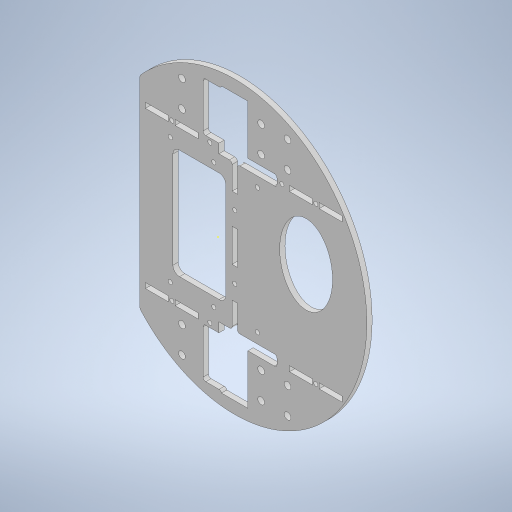
# Autodesk Inventor part: нижний эллипс тела
Saved by Autodesk Inventor 2023.1 (Build 271208000, 208)
## iProperties
Created: 2024-11-21
Part Number: нижний эллипс тела
Material: Типовые
Document SubType Name: Modeling
Designer: DELL
Density: 1 g/cm^3
Appearance: По умолчанию
Mass: 110.584 g
Surface Area: 588.358 cm^2
Volume: 110.584 cm^3
Author: DELL
Autodesk Inventor part; units mm, degrees
ref_plane "YZ Plane" through (0, 0, 0) normal (1, 0, 0) x (0, 1, 0)
ref_plane "XZ Plane" through (0, 0, 0) normal (0, 1, 0) x (-1, 0, 0)
ref_plane "XY Plane" through (0, 0, 0) normal (0, 0, 1) x (1, 0, 0)
sketch "Эскиз1" plane through (0, 0, 0) normal (0, 0, 1) x (1, 0, 0)
  ellipse E0 centre (12.6725, 0) end of major axis (12.6725, -110) minor radius 100
  dimension "d54" = 110
  dimension "d55" = 100
  constraints: 2 other
extrude "Выдавливание1" add sketch "Эскиз1" against normal blind 4
sketch "Эскиз5" plane through (0, 0, 0) normal (0, 0, 1) x (1, 0, 0)
  line L0 (10.6728, -60.9593) -> (10.6728, 60.5004) construction
  line L1 (14.6722, 60.5004) -> (14.6722, -60.9593) construction
  line L2 (14.6722, 60.5004) -> (10.6728, 60.5004)
  line L3 (14.6722, -60.9593) -> (10.6728, -60.9593)
  line L4 (10.6728, -35.9593) -> (14.6722, -35.9593)
  line L5 (10.6728, -12.5) -> (14.6722, -12.5)
  line L6 (10.6728, 12.5) -> (14.6722, 12.5)
  line L7 (10.6728, 35.5004) -> (14.6722, 35.5004)
  line L8 (10.6728, -12.5) -> (10.6728, 12.5)
  line L9 (14.6722, 12.5) -> (14.6722, -12.5)
  line L10 (14.6722, -12.5) -> (10.6728, 12.5) construction
  line L11 (10.6728, -60.9593) -> (10.6728, -35.9593)
  line L12 (14.6722, -35.9593) -> (14.6722, -60.9593)
  line L13 (14.6722, 35.5004) -> (14.6722, 60.5004)
  line L14 (10.6728, 35.5004) -> (10.6728, 60.5004)
  line L15 (14.6722, -35.9593) -> (10.6728, -12.5) construction
  circle A0 centre (12.6725, -24.2296) radius 1.575
  line L16 (14.6722, 12.5) -> (10.6728, 35.5004) construction
  circle A1 centre (12.6725, 24.0002) radius 1.575
  point P0 (0, 0)
  point P1 (12.6725, 0)
  point P2 (12.6725, 60.5004)
  point P3 (12.6725, 12.5)
  point P4 (12.6725, -12.5)
  point P5 (12.6725, 0)
  dimension "d35" = 25
  dimension "d36" = 25
  dimension "d37" = 25
  dimension "d38" = 3.15
  dimension "d39" = 3.15
  constraints: 34 end point, 8 point on line, 6 midpoint, 4 collinear, 4 perpendicular, 2 centre point, 2 parallel, 1 coincident
  measures "d35" distance from line of L1.end L4
  measures "d36" vertical distance of point (12.673, 60.5) L7.end
  measures "d37" distance of point (12.673, 12.5) point (12.673, -12.5)
  measures "d38" diameter of A0
  measures "d39" diameter of A1
extrude "Выдавливание3" cut sketch "Эскиз5" against normal blind 4
sketch "Эскиз7" plane through (0, 0, 0) normal (0, 0, 1) x (1, 0, 0)
  line L0 (4.1681, 100.5004) -> (8.7181, 100.5004) projected
  line L1 (2.6681, 94.4504) -> (2.6681, 99.0004) projected
  line L2 (2.6681, -99.4593) -> (2.6681, -94.9093) projected
  line L3 (8.7181, -100.9593) -> (4.1681, -100.9593) projected
  line L4 (2.6681, 100.5004) -> (22.6681, 100.5004)
  line L5 (22.6681, 100.5004) -> (22.6681, 60.5004)
  line L6 (22.6681, 60.5004) -> (2.6681, 60.5004)
  line L7 (2.6681, 60.5004) -> (2.6681, 100.5004)
  line L8 (2.6681, -100.9593) -> (22.6681, -100.9593)
  line L9 (22.6681, -100.9593) -> (22.6681, -60.9593)
  line L10 (22.6681, -60.9593) -> (2.6681, -60.9593)
  line L11 (2.6681, -60.9593) -> (2.6681, -100.9593)
  circle A0 centre (-7.3319, 80.5004) radius 5
  circle A1 centre (-7.3319, -80.9593) radius 5
  point P0 (0, 0)
  point P1 (2.6681, 80.5004)
  point P2 (2.6681, -80.9593)
  dimension "d44" = 20
  dimension "d45" = 40
  dimension "d46" = 20
  dimension "d47" = 40
  dimension "d48" = 10
  dimension "d49" = 10
  dimension "d50" = 10
  dimension "d51" = 10
  constraints: 16 end point, 4 parallel, 2 centre point, 2 horizontal, 2 midpoint, 2 perpendicular, 1 point on line
  measures "d44" distance of L5.end L6.end
  measures "d45" distance of L4.end L5.end
  measures "d46" distance of L10.end L9.end
  measures "d47" distance of L9.end L8.end
  measures "d48" diameter of A0
  measures "d49" diameter of A1
  measures "d50" distance of point (2.668, 80.5) A0.centre
  measures "d51" distance of point (2.668, -80.959) A1.centre
extrude "Выдавливание4" cut sketch "Эскиз7" against normal blind 4 contours L0 L4 L5 L6 L7 L1 | L2 L11 L10 L9 L8 L3
sketch "Эскиз8" plane through (0, 0, 0) normal (0, 0, 1) x (1, 0, 0)
  line L0 (-1.3319, 62.0004) -> (-1.3319, 99.0004) construction
  line L1 (-1.3319, 99.0004) -> (-9.3319, 99.0004) projected
  arc A0 (-9.3319, 99.0004) -> (-11.3319, 97.0004) centre (-9.3319, 97.0004) ccw projected
  line L2 (-11.3319, 97.0004) -> (-11.3319, 64.0004) projected
  line L3 (-9.3319, 62.0004) -> (-1.3319, 62.0004) projected
  arc A1 (-11.3319, 64.0004) -> (-9.3319, 62.0004) centre (-9.3319, 64.0004) ccw projected
  line L4 (-1.3319, -62.4593) -> (-9.3319, -62.4593) projected
  line L5 (-1.3319, -99.4593) -> (-1.3319, -62.4593) construction
  arc A2 (-9.3319, -62.4593) -> (-11.3319, -64.4593) centre (-9.3319, -64.4593) ccw projected
  line L6 (-11.3319, -64.4593) -> (-11.3319, -97.4593) projected
  line L7 (-9.3319, -99.4593) -> (-1.3319, -99.4593) projected
  arc A3 (-11.3319, -97.4593) -> (-9.3319, -99.4593) centre (-9.3319, -97.4593) ccw projected
  line L8 (-1.3319, -62.4593) -> (2.6681, -62.4593)
  line L9 (2.6681, -100.9593) -> (2.6681, -60.9593) construction
  line L10 (-1.3319, -99.4593) -> (2.6681, -99.4593)
  line L11 (2.6681, -60.9593) -> (2.6681, -100.9593) construction
  line L12 (2.6681, 60.5004) -> (2.6681, 100.5004) construction
  line L13 (-1.3319, 99.0004) -> (2.6681, 99.0004)
  line L14 (2.6681, 61.8452) -> (2.6681, 99.0004)
  line L15 (2.6681, -99.4593) -> (2.6681, -62.4593)
  line L16 (-1.3319, 62.0004) -> (2.6681, 62.0004)
  constraints: 12 end point, 4 point on line, 2 collinear, 2 horizontal, 1 parallel, 1 perpendicular
extrude "Выдавливание5" cut sketch "Эскиз8" against normal blind 10
fillet "Сопряжение1" radius 2 4 edges at (2.6681, -99.4593, -2) (2.6681, -62.4593, -2) (2.6681, 99.0004, -2) (2.6681, 62.0004, -2)
sketch "Эскиз11" plane through (0, 0, 0) normal (0, 0, 1) x (1, 0, 0)
  line L0 (-57.6761, -50.5044) -> (-57.6752, -40.5044) construction
  line L1 (-57.6682, 40.4956) -> (-57.6673, 50.4956) construction
  line L2 (-34.1607, 42.5053) -> (-34.1629, 17.1284) projected
  line L3 (-34.1658, -17.1413) -> (-34.168, -42.5182) projected
  line L4 (-29.1607, 42.5053) -> (0.8393, 42.5053)
  line L5 (5.8393, 37.5053) -> (5.8393, -35.5064)
  line L6 (0.8393, -40.5064) -> (-29.1607, -40.5064)
  line L7 (-34.1607, -35.5064) -> (-34.1607, 37.5053)
  arc A0 (5.8393, 37.5053) -> (0.8393, 42.5053) centre (0.8393, 37.5053) ccw
  arc A1 (-29.1607, 42.5053) -> (-34.1607, 37.5053) centre (-29.1607, 37.5053) ccw
  arc A2 (0.8393, -40.5064) -> (5.8393, -35.5064) centre (0.8393, -35.5064) ccw
  arc A3 (-34.1607, -35.5064) -> (-29.1607, -40.5064) centre (-29.1607, -35.5064) ccw
  point P0 (5.8393, -40.5064)
  point P1 (-34.1644, 37.5186)
  point P2 (-34.1644, 17.1349)
  point P3 (-34.1644, -17.1347)
  point P4 (-34.1643, -35.5283)
  dimension "d62" = 5
  constraints: 8 end point, 8 point on circle, 8 tangent, 4 centre point, 4 point on line, 3 equal radius, 2 parallel, 1 horizontal, 1 perpendicular
  measures "d62" radius of A0
extrude "Выдавливание6" cut sketch "Эскиз11" against normal blind 10
sketch "Эскиз13" plane through (0, 0, -4) normal (0, 0, -1) x (-1, 0, 0)
  circle A0 centre (36.1684, -47.5062) radius 1.5999 projected
  circle A1 centre (36.1601, 47.4937) radius 1.5999 projected
  circle A2 centre (36.1685, -47.5063) radius 1.5999 projected
  circle A3 centre (3.1684, -47.5091) radius 1.6001 projected
  circle A4 centre (3.1602, 47.4909) radius 1.6 projected
  circle A5 centre (36.1603, 47.4938) radius 1.6001 projected
  circle A6 centre (36.1602, 47.4937) radius 1.6 projected
  circle A7 centre (3.1602, 47.4909) radius 1.6001 projected
  circle A8 centre (-29.8398, 47.488) radius 1.6 projected
  circle A9 centre (-29.8314, -47.512) radius 1.5999 projected
  point P0 (0, 0)
extrude "Выдавливание7" cut sketch "Эскиз13" against normal blind 10
sketch "Эскиз14" plane through (0, 0, 0) normal (0, 0, 1) x (1, 0, 0)
  ellipse E0 centre (12.6725, 0) end of major axis (12.6725, -110) minor radius 100 construction
  line L0 (-59.1644, -35.4999) -> (-59.1644, 37.5118) construction
  line L1 (-59.1644, -76.5229) -> (-59.1644, 141.0841)
  ellipse E1 centre (12.6725, 0) end of major axis (12.6725, -110) minor radius 100 projected
  arc A0 (-59.1644, 76.5229) -> (-59.1644, -76.5229) centre (-11.9429, 0) ccw
  point P0 (0, 0)
  point P1 (-59.1644, 1.006)
  constraints: 4 end point, 2 point on circle, 2 point on line, 1 centre point, 1 midpoint, 1 vertical, 4 other
extrude "Выдавливание8" cut sketch "Эскиз14" against normal blind 10 contours E1 L1 picked at (-68.469, -2.5871)
fillet "Сопряжение2" radius 3 2 edges at (-59.1644, -76.5229, -2) (-59.1644, 76.5229, -2)
sketch "Эскиз15" plane through (0, 0, -4) normal (0, 0, -1) x (-1, 0, 0)
  line L0 (-42.6669, 57.0001) -> (-42.6669, 61.0001) construction
  line L1 (-42.6669, 61.0001) -> (-2.6669, 61.0001) construction
  line L2 (-2.6669, 61.0001) -> (-2.6669, 57.0001) construction
  line L3 (-2.6669, 57.0001) -> (-42.6669, 57.0001) construction
  line L4 (-42.6684, -61.2294) -> (-42.6683, -57.2294) construction
  line L5 (-42.6683, -57.2294) -> (-2.6683, -57.2296) construction
  line L6 (-2.6683, -57.2296) -> (-2.6684, -61.2296) construction
  line L7 (-2.6684, -61.2296) -> (-42.6684, -61.2294) construction
  line L8 (-44.6669, 55.0001) -> (-44.6669, 63.0001)
  line L9 (-44.6669, 63.0001) -> (-0.6669, 63.0001)
  line L10 (-0.6669, 63.0001) -> (-0.6669, 55.0001)
  line L11 (-0.6669, 55.0001) -> (-44.6669, 55.0001)
  line L12 (-44.6684, -63.2294) -> (-44.6683, -55.2294)
  line L13 (-44.6683, -55.2294) -> (-0.6683, -55.2296)
  line L14 (-0.6683, -55.2296) -> (-0.6684, -63.2296)
  line L15 (-0.6684, -63.2296) -> (-44.6684, -63.2294)
  point P0 (0, 0)
  dimension "d72" = 2
  dimension "d73" = 2
  constraints: 32 end point, 6 other
  measures "d72" distance between parallel lines of L3 L11
  measures "d73" distance between parallel lines of L7 L15
extrude "Выдавливание9" cut sketch "Эскиз15" against normal blind 10
fillet "Сопряжение3" radius 2 8 edges at (44.6669, 63.0001, -2) (44.6669, 55.0001, -2) (14.6722, 55.0001, -2) (10.6728, 55.0001, -2) (44.6683, -55.2294, -2) (44.6684, -63.2294, -2) (14.6722, -55.2296, -2) (10.6728, -55.2296, -2)
sketch "Эскиз16" plane through (0, 0, 0) normal (0, 0, 1) x (1, 0, 0)
  ellipse E0 centre (66.7121, 15.5627) end of major axis (66.7121, 45.5627) minor radius 20
  point P0 (0, 0)
  dimension "d84" = 30
  dimension "d85" = 20
  constraints: 2 other
extrude "Выдавливание10" cut sketch "Эскиз16" against normal blind 10
sketch "Эскиз17" plane through (0, 0, 0) normal (0, 0, 1) x (1, 0, 0)
  line L0 (-54.9896, -57.2298) -> (-54.9896, -61.2298) projected
  line L1 (-37.4896, -61.2298) -> (-37.4896, -57.2298) projected
  line L2 (-54.9896, -61.2298) -> (-37.4896, -61.2298) projected
  line L3 (-37.4896, -57.2298) -> (-54.9896, -57.2298) projected
  line L4 (-14.9896, -61.2297) -> (-14.9896, -57.2297) projected
  line L5 (-32.4896, -61.2298) -> (-14.9896, -61.2297) projected
  line L6 (-32.4896, -57.2298) -> (-32.4896, -61.2298) projected
  line L7 (-14.9896, -57.2297) -> (-32.4896, -57.2298) projected
extrude "Выдавливание11" cut sketch "Эскиз17" against normal blind 10 contours L3 L1 L2 L0
sketch "Эскиз18" plane through (0, 0, 0) normal (0, 0, 1) x (1, 0, 0)
  line L0 (76.6248, 61) -> (94.1248, 61)
  line L1 (94.1248, 57) -> (76.6248, 57)
  line L2 (76.6248, 57) -> (76.6248, 61)
  line L3 (54.1248, 61.0001) -> (71.6248, 61)
  line L4 (71.6248, 61) -> (71.6248, 57)
  line L5 (-54.9911, 61.0001) -> (-37.4911, 61.0001)
  line L6 (-37.4911, 61.0001) -> (-37.4911, 57.0001)
  line L7 (94.1263, -57.2292) -> (76.6263, -57.2293)
  line L8 (76.6263, -57.2293) -> (76.6263, -61.2293)
  line L9 (71.6263, -61.2293) -> (71.6263, -57.2293)
  line L10 (71.6263, -57.2293) -> (54.1263, -57.2294)
  line L11 (-37.4911, 57.0001) -> (-54.9911, 57.0001)
  line L12 (-54.9911, 57.0001) -> (-54.9911, 61.0001)
  line L13 (-32.4911, 61.0001) -> (-32.4911, 57.0001)
  line L14 (-32.4911, 61.0001) -> (-37.4911, 57.0001) construction
  circle A0 centre (-34.9911, 59.0001) radius 1.575
  line L15 (-32.4896, -61.2298) -> (-32.4896, -57.2298)
  line L16 (-14.9896, -57.2297) -> (-14.9896, -61.2297)
  line L17 (-14.9911, 57.0001) -> (-14.9911, 61.0001)
  line L18 (-14.9911, 61.0001) -> (-32.4911, 61.0001)
  line L19 (-32.4911, 57.0001) -> (-14.9911, 57.0001)
  line L20 (-14.9896, -57.2297) -> (-32.4896, -57.2298)
  line L21 (-32.4896, -61.2298) -> (-14.9896, -61.2297)
  line L22 (-37.4896, -57.2298) -> (-37.4896, -61.2298) construction
  line L23 (-32.4896, -61.2298) -> (-37.4896, -57.2298) construction
  circle A1 centre (-34.9896, -59.2298) radius 1.575
  line L24 (54.1248, 61.0001) -> (54.1248, 57.0001)
  line L25 (71.6248, 57) -> (54.1248, 57.0001)
  line L26 (94.1248, 57) -> (94.1248, 61)
  line L27 (76.6248, 57) -> (71.6248, 61) construction
  circle A2 centre (74.1248, 59) radius 1.575
  line L28 (-4.5856, -57.2296) -> (-4.5856, -61.2296) construction
  line L29 (-7.7356, -61.2297) -> (-7.7356, -57.2297) construction
  line L30 (-4.5856, -61.2296) -> (-7.7356, -57.2297) construction
  circle A3 centre (-6.1606, -59.2296) radius 1.575
  line L31 (-4.5871, 57.0001) -> (-4.5871, 61.0001) construction
  line L32 (-7.7371, 61.0001) -> (-7.7371, 57.0001) construction
  line L33 (-4.5871, 57.0001) -> (-7.7371, 61.0001) construction
  circle A4 centre (-6.1621, 59.0001) radius 1.575
  line L34 (49.9708, 57.0001) -> (49.9708, 61.0001) construction
  line L35 (46.8208, 61.0001) -> (46.8208, 57.0001) construction
  line L36 (49.9708, 57.0001) -> (46.8208, 61.0001) construction
  circle A5 centre (48.3958, 59.0001) radius 1.575
  line L37 (76.6263, -61.2293) -> (94.1263, -61.2293)
  line L38 (94.1263, -61.2293) -> (94.1263, -57.2292)
  line L39 (71.6263, -61.2293) -> (54.1263, -61.2293)
  line L40 (54.1263, -61.2293) -> (54.1263, -57.0459)
  line L41 (76.6263, -61.2293) -> (71.5581, -57.2293) construction
  circle A6 centre (74.0922, -59.2293) radius 1.575
  point P0 (0, 0)
  point P1 (54.1263, -57.2294)
  dimension "d88" = 3.15
  dimension "d90" = 3.15
  dimension "d91" = 3.15
  dimension "d92" = 3.15
  dimension "d93" = 3.15
  dimension "d94" = 3.15
  dimension "d95" = 3.15
  constraints: 84 end point, 7 centre point, 7 midpoint, 6 perpendicular, 2 horizontal, 2 parallel, 1 point on line
  measures "d88" diameter of A0
  measures "d90" diameter of A1
  measures "d91" diameter of A2
  measures "d92" diameter of A3
  measures "d93" diameter of A4
  measures "d94" diameter of A5
  measures "d95" diameter of A6
extrude "Выдавливание12" cut sketch "Эскиз18" against normal blind 10
sketch "Эскиз19" plane through (0, 0, -4) normal (0, 0, -1) x (-1, 0, 0)
  circle A0 centre (-32.6681, -90.9593) radius 2.55 projected
  circle A1 centre (-32.6681, -70.9593) radius 2.55 projected
  circle A2 centre (-52.6681, -90.9593) radius 2.55 projected
  circle A3 centre (-52.6681, -70.9593) radius 2.55 projected
  circle A4 centre (27.3319, -90.9593) radius 2.55 projected
  circle A5 centre (27.3319, -70.9593) radius 2.55 projected
  circle A6 centre (-52.6681, 70.5004) radius 2.55 projected
  circle A7 centre (-52.6681, 90.5004) radius 2.55 projected
  circle A8 centre (-32.6681, 70.5004) radius 2.55 projected
  circle A9 centre (-32.6681, 90.5004) radius 2.55 projected
  circle A10 centre (27.3319, 90.5004) radius 2.55 projected
  circle A11 centre (27.3319, 70.5004) radius 2.55 projected
  point P0 (0, 0)
extrude "Выдавливание13" cut sketch "Эскиз19" against normal blind 10
sketch "Эскиз20" plane through (0, 0, 0) normal (0, 0, 1) x (1, 0, 0)
  point P0 (0, 0)
